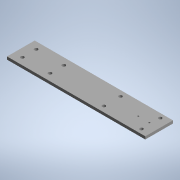
# Autodesk Inventor part: adapter_chipshouter
Saved by Autodesk Inventor 2022 (Build 260153000, 153)
## iProperties
Part Number: adapter_chipshouter
Material: Allgemein
Document SubType Name: Modellieren
Designer: Niclas
Appearance: Vorgabe
Author: Niclas
Autodesk Inventor part; units mm, degrees
ref_plane "YZ-Ebene" through (0, 0, 0) normal (1, 0, 0) x (0, 1, 0)
ref_plane "XZ-Ebene" through (0, 0, 0) normal (0, 1, 0) x (-1, 0, 0)
ref_plane "XY-Ebene" through (0, 0, 0) normal (0, 0, 1) x (1, 0, 0)
sketch "Skizze1" plane through (0, 0, 0) normal (0, 1, 0) x (-1, 0, 0)
  line L0 (250, -50) -> (0, -50)
  line L1 (0, -50) -> (0, 0)
  line L2 (0, 0) -> (250, 0)
  line L3 (250, 0) -> (250, -50)
  dimension "d0" = 250
  dimension "d1" = 50
  constraints: 8 end point, 2 parallel, 1 coincident, 1 horizontal, 1 perpendicular
  measures "d0" distance of L0.start L0.end
  measures "d1" distance of L2.end L0.start
extrude "Extrusion1" add sketch "Skizze1" along normal blind 5
sketch "Skizze2" plane through (0, 5, 0) normal (0, 1, 0) x (1, 0, 0)
  circle A0 centre (-235, 37.5) radius 3.1
  circle A1 centre (-185, 37.5) radius 3.1
  circle A2 centre (-235, 12.5) radius 3.1
  circle A3 centre (-185, 12.5) radius 3.1
  line L0 (0, 50) -> (-250, 50) projected
  line L1 (-250, 50) -> (-250, 0) projected
  point P0 (0, 0)
  dimension "d4" = 6.2
  dimension "d5" = 6.2
  dimension "d6" = 6.2
  dimension "d7" = 6.2
  dimension "d8" = 12.5
  dimension "d9" = 25
  dimension "d10" = 25
  dimension "d11" = 50
  dimension "d12" = 50
  dimension "d13" = 15
  dimension "d14" = 15
  dimension "d15" = 12.5
  constraints: 4 centre point
  measures "d4" diameter of A0
  measures "d5" diameter of A1
  measures "d6" diameter of A3
  measures "d7" diameter of A2
  measures "d8" distance from line of L0 A0.centre
  measures "d9" distance of A2.centre A0.centre
  measures "d10" distance of A3.centre A1.centre
  measures "d11" distance of A0.centre A1.centre
  measures "d12" distance of A3.centre A2.centre
  measures "d13" distance from line of L1 A0.centre
  measures "d14" distance from line of L1 A2.centre
  measures "d15" distance from line of L0 A1.centre
extrude "Extrusion2" cut sketch "Skizze2" against normal blind 6
sketch "Skizze3" plane through (0, 5, 0) normal (0, 1, 0) x (1, 0, 0)
  circle A0 centre (-15, 42) radius 3
  circle A1 centre (-15, 8) radius 3
  circle A2 centre (-84.9714, 10) radius 3
  circle A3 centre (-85, 40) radius 3
  line L0 (0, 0) -> (0, 50) projected
  line L1 (0, 50) -> (-250, 50) projected
  dimension "d18" = 6
  dimension "d19" = 6
  dimension "d20" = 6
  dimension "d21" = 6
  dimension "d22" = 15
  dimension "d23" = 15
  dimension "d24" = 70
  dimension "d25" = 70
  dimension "d26" = 34
  dimension "d27" = 30
  dimension "d28" = 10
  dimension "d29" = 8
  constraints: 4 centre point
  measures "d18" diameter of A3
  measures "d19" diameter of A0
  measures "d20" diameter of A1
  measures "d21" diameter of A2
  measures "d22" distance from line of L0 A1.centre
  measures "d23" distance from line of L0 A0.centre
  measures "d24" horizontal distance of A0.centre A3.centre
  measures "d25" distance of A2.centre A1.centre
  measures "d26" distance of A1.centre A0.centre
  measures "d27" distance of A2.centre A3.centre
  measures "d28" distance from line of L1 A3.centre
  measures "d29" distance from line of L1 A0.centre
extrude "Extrusion3" cut sketch "Skizze3" against normal blind 10
sketch "Skizze4" plane through (0, 5, 0) normal (0, 1, 0) x (1, 0, 0)
  circle A0 centre (-38, 25) radius 1.5
  circle A1 centre (-18, 25) radius 1.5
  line L0 (0, 50) -> (-250, 50) projected
  line L1 (0, 0) -> (0, 50) projected
  dimension "d32" = 3
  dimension "d33" = 3
  dimension "d34" = 25
  dimension "d35" = 25
  dimension "d36" = 18
  dimension "d37" = 20
  constraints: 2 centre point
  measures "d32" diameter of A0
  measures "d33" diameter of A1
  measures "d34" distance from line of L0 A1.centre
  measures "d35" distance from line of L0 A0.centre
  measures "d36" distance from line of L1 A1.centre
  measures "d37" distance of A1.centre A0.centre
extrude "Extrusion4" cut sketch "Skizze4" against normal blind 10
